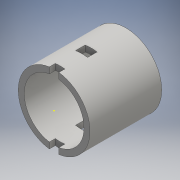
# Autodesk Inventor part: pipe
Saved by Autodesk Inventor 2016 (Build 200138000, 138)
## iProperties
Created: 2016-05-12
Part Number: pipe
Material: 一般
Document SubType Name: Modeling
Designer: 宏太
Density: 1 g/cm^3
Appearance: 既定
Author: 宏太
Autodesk Inventor part; units mm, degrees
ref_plane "YZ Plane" through (0, 0, 0) normal (1, 0, 0) x (0, 1, 0)
ref_plane "XZ Plane" through (0, 0, 0) normal (0, 1, 0) x (-1, 0, 0)
ref_plane "XY Plane" through (0, 0, 0) normal (0, 0, 1) x (1, 0, 0)
sketch "スケッチ1" plane through (0, 0, 0) normal (0, 1, 0) x (-1, 0, 0)
  circle A0 centre (0, 0) radius 25
  circle A1 centre (0, 0) radius 30
  dimension "d0" = 50
  dimension "d1" = 60
  constraints: 2 centre point, 2 coincident
  measures "d0" diameter of A0
  measures "d1" diameter of A1
extrude "押し出し1" add sketch "スケッチ1" along normal blind 60
sketch "スケッチ2" plane through (0, 0, 0) normal (0, 0, 1) x (1, 0, 0)
  line L0 (-5, 30.9364) -> (5, 30.9364)
  line L1 (5, 30.9364) -> (5, 22.9364)
  line L2 (5, 22.9364) -> (-5, 22.9364)
  line L3 (-5, 22.9364) -> (-5, 30.9364)
  line L4 (-5, 30.9364) -> (5, 22.9364) construction
  line L5 (5, 30.9364) -> (-5, 22.9364) construction
  point P0 (0, 0)
  point P1 (0, 26.9364)
  dimension "d4" = 10
  dimension "d5" = 8
  constraints: 12 end point, 2 midpoint, 2 parallel, 1 horizontal, 1 perpendicular
  measures "d4" distance of L1.end L2.end
  measures "d5" distance of L0.end L1.end
extrude "押し出し2" cut sketch "スケッチ2" along normal mid plane 60
sketch "スケッチ3" plane through (0, 0, 0) normal (0, 0, 1) x (1, 0, 0)
  point P0 (0, 0)
sketch "スケッチ4" plane through (0, 0, 0) normal (0, 0, 1) x (1, 0, 0)
  line L0 (4, -5) -> (-4, -5)
  line L1 (-4, -5) -> (-4, 5)
  line L2 (-4, 5) -> (4, 5)
  line L3 (4, 5) -> (4, -5)
  line L4 (4, -5) -> (-4, 5) construction
  line L5 (-4, -5) -> (4, 5) construction
  point P0 (0, 0)
  dimension "d8" = 8
  dimension "d9" = 10
  constraints: 12 end point, 2 midpoint, 2 parallel, 1 horizontal, 1 perpendicular
  measures "d8" distance of L1.end L2.end
  measures "d9" distance of L0.end L1.end
extrude "押し出し3" cut sketch "スケッチ4" along normal mid plane 60
